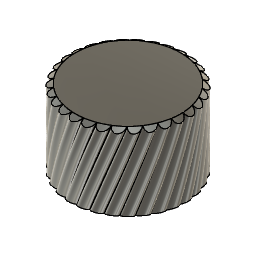
duckypad_pro_knob_fusion360 (Autodesk Fusion 360 design; units mm, degrees)
Autodesk Fusion 360 part; units mm, degrees
sketch "Sketch1" plane through (0, 0, 0) normal (0, 0, 1) x (1, 0, 0)
  circle A0 centre (0, 0) radius 7.5
  circle A1 centre (0, 0) radius 7.5 construction
  arc A2 (1.2146, 7.401) -> (-0.2806, 7.4948) centre (0.4694, 7.4853) ccw
  arc A3 (-0.3507, 7.4918) -> (-1.8327, 7.2726) centre (-1.0972, 7.4193) ccw
  arc A4 (-1.9006, 7.2552) -> (-3.3047, 6.7327) centre (-2.6157, 7.0291) ccw
  arc A5 (-3.3675, 6.7015) -> (-4.6323, 5.8985) centre (-4.02, 6.3316) ccw
  arc A6 (-4.6873, 5.8549) -> (-5.7574, 4.8065) centre (-5.2486, 5.3575) ccw
  arc A7 (-5.8021, 4.7524) -> (-6.6309, 3.5044) centre (-6.2478, 4.1491) ccw
  arc A8 (-6.6634, 3.4422) -> (-7.2146, 2.0492) centre (-6.9739, 2.7595) ccw
  arc A9 (-7.2335, 1.9816) -> (-7.483, 0.5044) centre (-7.3952, 1.2492) ccw
  arc A10 (-7.4874, 0.4344) -> (-7.4244, -1.0624) centre (-7.4934, -0.3156) ccw
  arc A11 (-7.4141, -1.1319) -> (-7.0412, -2.5828) centre (-7.264, -1.8667) ccw
  arc A12 (-7.0168, -2.6486) -> (-6.3504, -3.9903) centre (-6.7171, -3.3362) ccw
  arc A13 (-6.3128, -4.0496) -> (-5.382, -5.2235) centre (-5.8767, -4.6598) ccw
  arc A14 (-5.3328, -5.2736) -> (-4.1783, -6.2283) centre (-4.7795, -5.7798) ccw
  arc A15 (-4.1199, -6.2671) -> (-2.7921, -6.9609) centre (-3.4733, -6.6472) ccw
  arc A16 (-2.7268, -6.9867) -> (-1.2838, -7.3893) centre (-2.0154, -7.2241) ccw
  arc A17 (-1.2146, -7.401) -> (0.2806, -7.4948) centre (-0.4694, -7.4853) ccw
  arc A18 (0.3507, -7.4918) -> (1.8327, -7.2726) centre (1.0972, -7.4193) ccw
  arc A19 (1.9006, -7.2552) -> (3.3047, -6.7327) centre (2.6157, -7.0291) ccw
  arc A20 (3.3675, -6.7015) -> (4.6323, -5.8985) centre (4.02, -6.3316) ccw
  arc A21 (4.6873, -5.8549) -> (5.7574, -4.8065) centre (5.2486, -5.3575) ccw
  circle A22 centre (0, 0) radius 3
  line L0 (0, 0) -> (0, 1.5) construction
  line L1 (2.5981, 1.5) -> (-2.5981, 1.5)
  arc A23 (5.8021, -4.7524) -> (6.6309, -3.5044) centre (6.2478, -4.1491) ccw
  arc A24 (6.6634, -3.4422) -> (7.2146, -2.0492) centre (6.9739, -2.7595) ccw
  arc A25 (7.2335, -1.9816) -> (7.483, -0.5044) centre (7.3952, -1.2492) ccw
  arc A26 (7.4874, -0.4344) -> (7.4244, 1.0624) centre (7.4934, 0.3156) ccw
  arc A27 (7.4141, 1.1319) -> (7.0412, 2.5828) centre (7.264, 1.8667) ccw
  arc A28 (7.0168, 2.6486) -> (6.3504, 3.9903) centre (6.7171, 3.3362) ccw
  arc A29 (6.3128, 4.0496) -> (5.382, 5.2235) centre (5.8767, 4.6598) ccw
  arc A30 (5.3328, 5.2736) -> (4.1783, 6.2283) centre (4.7795, 5.7798) ccw
  arc A31 (4.1199, 6.2671) -> (2.7921, 6.9609) centre (3.4733, 6.6472) ccw
  arc A32 (2.7268, 6.9867) -> (1.2838, 7.3893) centre (2.0154, 7.2241) ccw
  circle A33 centre (0, 0) radius 4.5
  dimension "d3" = 15
  dimension "d5" = 15
  dimension "d6" = 1.5
  dimension "d9" = 360
  dimension "d23" = 6
  dimension "d25" = 1.5
  constraint coincident A0.centre A1.centre
  constraint concentric A0 A1
  constraint coincident A1 A2.centre
  constraint coincident A0 A2.end
  constraint coincident A0 A2.start
  constraint concentric A1 A22
  constraint vertical L0
  constraint perpendicular L0 L1
  constraint coincident A22 L1.end
  constraint coincident A22 L1.start
  constraint coincident L0.end L1
  measures "d3" diameter of A0
  measures "d5" diameter of A1
  measures "d6" diameter of A2
  measures "d23" diameter of A22
  measures "d25" distance of A0.centre L0.end
sketch "Sketch3" plane through (0, 0, 0) normal (0, 1, 0) x (1, 0, 0)
  line L0 (0, 0) -> (0, -11)
  dimension "d29" = 11
  constraint coincident L0.start origin
  constraint vertical L0
  measures "d29" distance of L0.start L0.end
sweep "Sweep1" add twist angle 30 profiles "Sketch1" path "Sketch3" along L0 section 1 contours A0 | A0 A26 | A0 A27 | A0 A25 | A0 A28 | A0 A24 | A0 A29 | A0 A23 | A0 A30 | A0 A21 | A0 A31 | A0 A20 | A0 A32 | A0 A19 | A0 A2 | A0 A18 | A0 A3 | A0 A17 | A0 A4 | A0 A16 | A0 A5 | A0 A15 | A0 A6 | A0 A14 | A0 A7 | A0 A13 | A0 A8 | A0 A12 | A0 A9 | A0 A11 | A0 A10 | A22 L1 | A22 L1 | A33
sketch "Sketch2" plane through (0, 0, 0) normal (1, 0, 0) x (0, 1, 0)
  line L0 (0, 0) -> (7.5, 0) construction
  line L1 (7.5, 0) -> (10.0981, 1.5)
  line L2 (7.5, 0) -> (9, 0) construction
  line L3 (10.0981, 1.5) -> (10.0981, 0)
  line L4 (7.5, 0) -> (10.0981, 0)
  line L5 (0, 0) -> (0, 11) construction
  line L6 (0, 11) -> (7.5, 11)
  line L7 (7.5, 11) -> (10.0981, 9.5)
  line L8 (7.5, 11) -> (9, 11) construction
  line L9 (10.0981, 9.5) -> (10.0981, 11)
  line L10 (7.5, 11) -> (10.0981, 11)
  dimension "d12" = 7.5
  dimension "d13" = 30
  dimension "d14" = 3
  dimension "d17" = 11
  dimension "d18" = 7.5
  dimension "d19" = 3
  dimension "d20" = 30
  constraint coincident L0.start L5.start
  constraint horizontal L0
  constraint horizontal L2
  constraint coincident L2 L3.end
  constraint perpendicular L2 L3
  constraint perpendicular L0 L5
  constraint perpendicular L5 L6
  constraint horizontal L8
  constraint coincident L8 L9.end
  constraint perpendicular L8 L9
  measures "d12" distance of L0.start L0.end
  measures "d13" angle of L1 L2
  measures "d14" distance of L0.end L1.end
  measures "d17" distance of L0.start L5.end
  measures "d18" distance of L5.end L6.end
  measures "d19" distance of L6.end L7.end
  measures "d20" angle of L7 L8
revolve "Revolve4" cut sketch "Sketch2" angle 360 about axis through (0, 0, 0) along (0, 0, 1)
extrude "Extrude4" cut sketch "Sketch1" along normal blind 9 contours A22 L1 picked at (-0.5998, 0.0443)
extrude "Extrude6" cut sketch "Sketch1" along normal blind 4 contours A22 L1 | A33 picked at (-0.7492, 2.0593)
equation "knob_base_dia = 15 mm"
equation "knob_height = 11 mm"
equation "d3 = knob_base_dia"
equation "groove_dia = 1.5 mm"
equation "d5 = knob_base_dia"
equation "d6 = groove_dia"
equation "groove_count = 30"
equation "d8 = groove_count"
equation "d12 = knob_base_dia / 2"
equation "d13 = chamfer_degree"
equation "d14 = groove_dia * 2"
equation "chamfer_degree = 30 deg"
equation "d17 = knob_height"
equation "d18 = knob_base_dia / 2"
equation "d19 = groove_dia * 2"
equation "d20 = chamfer_degree"
equation "shaft_dia = ( 6 * shaft_factor ) * 1 mm"
equation "d23 = shaft_dia"
equation "D_length = 4.5 mm"
equation "d25 = shaft_dia - D_length"
equation "shaft_depth = 9 mm"
equation "d29 = knob_height"
equation "sweep_deg = 30 deg"
equation "d35 = sweep_deg"
equation "shaft_factor = 1"
equation "d42 = shaft_depth"
equation "base_step = 4 mm"
equation "d47 = ( knob_base_dia - shaft_dia )"
equation "d48 = base_step"
